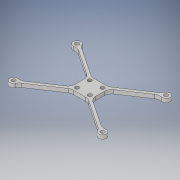
# Autodesk Inventor part: led_brace
Saved by Autodesk Inventor 2017 (Build 210142000, 142)
## iProperties
Created: 2017-06-15
Part Number: led_brace
Material: Generic
Document SubType Name: Modeling
Designer: millerid
Density: 1 g/cm^3
Appearance: Default
Author: millerid
Autodesk Inventor part; units mm, degrees
ref_plane "YZ Plane" through (0, 0, 0) normal (1, 0, 0) x (0, 1, 0)
ref_plane "XZ Plane" through (0, 0, 0) normal (0, 1, 0) x (-1, 0, 0)
ref_plane "XY Plane" through (0, 0, 0) normal (0, 0, 1) x (1, 0, 0)
sketch "Sketch1" plane through (0, 0, 0) normal (0, 1, 0) x (-1, 0, 0)
  circle A0 centre (4.9867, -4.611) radius 1.5
  circle A1 centre (75.1867, -4.611) radius 1.5
  circle A2 centre (4.9867, -54.611) radius 1.5
  circle A3 centre (75.1867, -54.611) radius 1.5
  circle A4 centre (45.1867, -24.611) radius 1.5
  circle A5 centre (34.9867, -24.611) radius 1.5
  circle A6 centre (45.1867, -34.611) radius 1.5
  circle A7 centre (34.9867, -34.611) radius 1.5
  line L0 (48.1982, -20.6033) -> (70.3378, -5.8436)
  line L1 (50.8585, -21.3298) -> (70.166, -8.4581)
  line L2 (50.8585, -37.8922) -> (70.166, -50.7639)
  line L3 (48.1982, -38.6187) -> (70.3378, -53.3784)
  line L4 (31.9751, -20.6033) -> (9.8356, -5.8436)
  line L5 (29.3149, -21.3298) -> (10.0074, -8.4581)
  line L6 (31.9751, -38.6187) -> (9.8702, -53.3553)
  line L7 (29.3149, -37.8922) -> (10.0529, -50.7336)
  line L8 (44.87, -21.611) -> (35.3033, -21.611)
  line L9 (31.9867, -26.3221) -> (31.9867, -32.8999)
  line L10 (35.3033, -37.611) -> (44.87, -37.611)
  arc A8 (31.9751, -20.6033) -> (35.3033, -21.611) centre (35.3033, -15.611) ccw
  arc A9 (44.87, -21.611) -> (48.1982, -20.6033) centre (44.87, -15.611) ccw
  line L11 (48.1867, -26.3221) -> (48.1867, -32.8999)
  arc A10 (50.8585, -21.3298) -> (48.1867, -26.3221) centre (54.1867, -26.3221) ccw
  arc A11 (48.1867, -32.8999) -> (50.8585, -37.8922) centre (54.1867, -32.8999) ccw
  arc A12 (48.1982, -38.6187) -> (44.87, -37.611) centre (44.87, -43.611) ccw
  arc A13 (35.3033, -37.611) -> (31.9751, -38.6187) centre (35.3033, -43.611) ccw
  arc A14 (29.3149, -37.8922) -> (31.9867, -32.8999) centre (25.9867, -32.8999) ccw
  arc A15 (31.9867, -26.3221) -> (29.3149, -21.3298) centre (25.9867, -26.3221) ccw
  arc A16 (74.6225, -7.5575) -> (72.461, -3.3578) centre (75.1867, -4.611) ccw
  arc A17 (72.461, -55.8643) -> (74.6225, -51.6645) centre (75.1867, -54.611) ccw
  arc A18 (5.5187, -51.6188) -> (7.7189, -55.9033) centre (4.8979, -54.6448) ccw
  arc A19 (7.7124, -3.3578) -> (5.5509, -7.5575) centre (4.9867, -4.611) ccw
  arc A20 (74.6225, -7.5575) -> (70.166, -8.4581) centre (73.4942, -13.4505) ccw
  arc A21 (70.3378, -5.8436) -> (72.461, -3.3578) centre (67.0096, -0.8513) ccw
  arc A22 (70.166, -50.7639) -> (74.6225, -51.6645) centre (73.4942, -45.7716) ccw
  arc A23 (72.461, -55.8643) -> (70.3378, -53.3784) centre (67.0096, -58.3707) ccw
  arc A24 (9.8702, -53.3553) -> (7.7189, -55.9033) centre (13.1984, -58.3476) ccw
  arc A25 (5.5187, -51.6188) -> (10.0529, -50.7336) centre (6.7247, -45.7413) ccw
  arc A26 (10.0074, -8.4581) -> (5.5509, -7.5575) centre (6.6792, -13.4505) ccw
  arc A27 (7.7124, -3.3578) -> (9.8356, -5.8436) centre (13.1638, -0.8513) ccw
  point P0 (0, 0)
  point P1 (72.1867, -4.611)
  point P2 (72.9454, -6.6052)
  point P3 (72.9454, -52.6168)
  point P4 (72.1867, -54.611)
  point P5 (7.9867, -4.611)
  point P6 (7.228, -6.6052)
  point P7 (7.9867, -54.611)
  point P8 (7.228, -52.6168)
  point P9 (7.228, -52.6168)
  dimension "d0" = 3
  dimension "d1" = 3
  dimension "d2" = 3
  dimension "d3" = 70.2
  dimension "d4" = 50
  dimension "d5" = 70.2
  dimension "d6" = 50
  dimension "d7" = 3
  dimension "d8" = 20
  dimension "d9" = 30
  dimension "d10" = 3
  dimension "d11" = 30
  dimension "d12" = 20
  dimension "d13" = 3
  dimension "d14" = 20
  dimension "d15" = 30
  dimension "d16" = 3
  dimension "d17" = 20
  dimension "d18" = 30
  dimension "d27" = 6
  dimension "d28" = 6
  dimension "d29" = 6
  constraints: 48 point on circle, 32 tangent, 28 centre point, 24 end point, 13 equal radius, 8 point on line, 4 parallel, 3 concentric, 2 perpendicular, 1 horizontal, 1 vertical
  measures "d0" diameter of A2
  measures "d1" diameter of A3
  measures "d2" diameter of A0
  measures "d3" distance of A1.centre A0.centre
  measures "d4" distance of A3.centre A1.centre
  measures "d5" distance of A2.centre A3.centre
  measures "d6" distance of A2.centre A0.centre
  measures "d7" diameter of A4
  measures "d8" vertical distance of A4.centre A1.centre
  measures "d9" horizontal distance of A4.centre A1.centre
  measures "d10" diameter of A5
  measures "d11" horizontal distance of A5.centre A0.centre
  measures "d12" vertical distance of A5.centre A0.centre
  measures "d13" diameter of A6
  measures "d14" vertical distance of A3.centre A6.centre
  measures "d15" horizontal distance of A6.centre A3.centre
  measures "d16" diameter of A7
  measures "d17" vertical distance of A2.centre A7.centre
  measures "d18" horizontal distance of A2.centre A7.centre
  measures "d27" radius of A8
  measures "d28" radius of A10
  measures "d29" radius of A20
extrude "Extrusion1" add sketch "Sketch1" along normal blind 3
equation "\"d11\" = d9"
equation "\"d12\" = d8"
equation "\"d14\" = d8"
equation "\"d15\" = d9"
equation "\"d17\" = d8"
equation "\"d18\" = d9"
body "Solid1"
